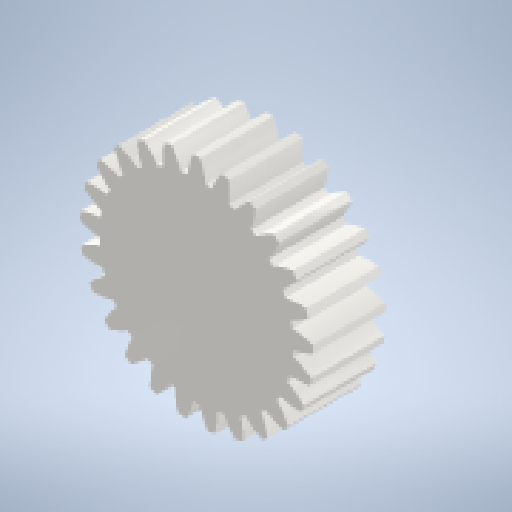
# Autodesk Inventor part: Spur Gear1
Saved by Autodesk Inventor 2023 (Build 270158030, 158C)
## iProperties
Created: 2024-09-26
Part Number: Spur Gear1
Material: Steel
Document SubType Name: Modeling
Designer: lvrectanus0
Categories: <?xml version="1.0" encoding="UTF-16"?> <MemberInstance><Categories><FamilyTemplate><FamilyTemplateParameter ValueType="xs:double" Id="1" ObjectReferenceKey="da_z" ObjectType="kUserParameterObject"/><FamilyTemplateParameter ValueType="xs:double" Id="2" ObjectReferenceKey="da_b" ObjectType="kUserParameterObject"/><FamilyTemplateParameter ValueType="xs:double" Id="3" ObjectReferenceKey="da_beta" ObjectType="kUserParameterObject"/><FamilyTemplateParameter ValueType="xs:double" Id="4" ObjectReferenceKey="da_da" ObjectType="kUserParameterObject"/><FamilyTemplateParameter ValueType="xs:double" Id="5" ObjectReferenceKey="da_aw" ObjectType="kUserParameterObject"/><FamilyTemplateParameter ValueType="xs:string" Id="6" ObjectReferenceKey="EAIAABAAAAC/AAAAAAAAAIAAAAAAAAAA" ObjectType="83910656" SubObjectId="SurfaceGeometry"/></FamilyTemplate><ParamToTemplateMap><ParamToTemplate CategoryParameter="//CategoryParameter[@InternalName='046C89C9-8512-4d59-83FE-43B91F4F132A']" TemplateParameter="1"/><ParamToTemplate CategoryParameter="//CategoryParameter[@InternalName='2552DF32-E462-4b46-AEBF-C6C7768E72AC']" TemplateParameter="2"/><ParamToTemplate CategoryParameter="//CategoryParameter[@InternalName='C9EE641D-15FC-4fae-A226-E94C4372FDD7']" TemplateParameter="3"/><ParamToTemplate><ParamToTemplate CategoryParameter="//CategoryParameter[@InternalName='00B6519A-459B-49c7-AD84-2E56D39A5744']" ConstantValue="0.000000"/></ParamToTemplate><ParamToTemplate><ParamToTemplate CategoryParameter="//CategoryParameter[@InternalName='04B31F0E-C7A6-4894-AA32-9629BEFACF47']" ConstantValue="1.000000"/></ParamToTemplate><ParamToTemplate><ParamToTemplate CategoryParameter="//CategoryParameter[@InternalName='43CBEC2E-7847-49e7-A936-2F7889FCB2D9']" ConstantValue="0.250000"/></ParamToTemplate><ParamToTemplate><ParamToTemplate CategoryParameter="//CategoryParameter[@InternalName='B1EFC894-105D-4ebd-86BF-FA20ED196853']" ConstantValue="0.350000"/></ParamToTemplate><ParamToTemplate><ParamToTemplate CategoryParameter="//CategoryParameter[@InternalName='51175063-3D10-4879-93E8-6246FE8B403D']" ConstantValue="2061532430.657340"/></ParamToTemplate><ParamToTemplate><ParamToTemplate CategoryParameter="//CategoryParameter[@InternalName='A3A52E27-4454-46a9-B0BD-C932399B70AF']" ConstantValue="0.300000"/></ParamToTemplate><ParamToTemplate><ParamToTemplate CategoryParameter="//CategoryParameter[@InternalName='91B76062-C214-41d9-B1B9-14D2AB99603D']" ConstantValue="0.149412"/></ParamToTemplate><ParamToTemplate><ParamToTemplate CategoryParameter="//CategoryParameter[@InternalName='374E806E-8B8A-4dda-A9AA-1039D6500AD2']" ConstantValue="6.692913"/></ParamToTemplate><ParamToTemplate><ParamToTemplate CategoryParameter="//CategoryParameter[@InternalName='2D373A89-B862-43d6-8D0B-0CBF12AB9F6C']" ConstantValue="0.349066"/></ParamToTemplate><ParamToTemplate CategoryParameter="//CategoryParameter[@InternalName='37777632-D6A2-4fac-9D53-DB8ACD95C989']" TemplateParameter="4"/><ParamToTemplate CategoryParameter="//CategoryParameter[@InternalName='FD1017F1-B727-4f7e-9707-0F86F1FF9423']" TemplateParameter="5"/><ParamToTemplate><ParamToTemplate CategoryParameter="//CategoryParameter[@InternalName='9E1B4470-B2D3-4ff1-B813-535BB4CDF51A']" ConstantValue="3523220.976809"/></ParamToTemplate><ParamToTemplate><ParamToTemplate CategoryParameter="//CategoryParameter[@InternalName='F8452263-BFF6-458c-9FB1-07C4B99E95CD']" ConstantValue="11397033.805607"/></ParamToTemplate><ParamToTemplate><ParamToTemplate CategoryParameter="//CategoryParameter[@InternalName='3E3BB259-FD49-497f-8171-6EBC954A3479']" ConstantValue="2.000000"/></ParamToTemplate><ParamToTemplate CategoryParameter="//CategoryParameter[@InternalName='27C3BAF2-7550-4e4b-AE2C-0DB134B7D9B7']" TemplateParameter="6"/></ParamToTemplateMap><Category DisplayName="Gear" InternalName="DC85795E-93AB-48d5-8EEE-5A27447B64BD" Mnemonic="Gear"><CategoryParameter DisplayName="z" InternalName="046C89C9-8512-4d59-83FE-43B91F4F132A" Mnemonic="z"/><CategoryParameter DisplayName="b" InternalName="2552DF32-E462-4b46-AEBF-C6C7768E72AC" Mnemonic="b"/><CategoryParameter DisplayName="||b|" InternalName="C9EE641D-15FC-4fae-A226-E94C4372FDD7" Mnemonic="beta"/><CategoryParameter DisplayName="x" InternalName="00B6519A-459B-49c7-AD84-2E56D39A5744" Mnemonic="x"/><CategoryParameter DisplayName="a*" InternalName="04B31F0E-C7A6-4894-AA32-9629BEFACF47" Mnemonic="a"/><CategoryParameter DisplayName="c*" InternalName="43CBEC2E-7847-49e7-A936-2F7889FCB2D9" Mnemonic="c"/><CategoryParameter DisplayName="r|.f|*" InternalName="B1EFC894-105D-4ebd-86BF-FA20ED196853" Mnemonic="rf"/><CategoryParameter DisplayName="E" InternalName="51175063-3D10-4879-93E8-6246FE8B403D" Mnemonic="E"/><CategoryParameter DisplayName="||m|" InternalName="A3A52E27-4454-46a9-B0BD-C932399B70AF" Mnemonic="mi"/><Category DisplayName="SpurGear" InternalName="26C5A22E-A91E-4dfd-A3B3-23CCAFAE1764" Mnemonic="SpurGear"><CategoryParameter DisplayName="m" InternalName="91B76062-C214-41d9-B1B9-14D2AB99603D" Mnemonic="m"/><CategoryParameter DisplayName="P" InternalName="374E806E-8B8A-4dda-A9AA-1039D6500AD2" Mnemonic="PP"/><CategoryParameter DisplayName="||a|" InternalName="2D373A89-B862-43d6-8D0B-0CBF12AB9F6C" Mnemonic="alpha"/><CategoryParameter DisplayName="d|.a|" InternalName="37777632-D6A2-4fac-9D53-DB8ACD95C989" Mnemonic="da"/><CategoryParameter DisplayName="a|.w|" InternalName="FD1017F1-B727-4f7e-9707-0F86F1FF9423" Mnemonic="aw"/><CategoryParameter DisplayName="||s||.Flim|" InternalName="9E1B4470-B2D3-4ff1-B813-535BB4CDF51A" Mnemonic="sFlim"/><CategoryParameter DisplayName="||s||.Hlim|" InternalName="F8452263-BFF6-458c-9FB1-07C4B99E95CD" Mnemonic="sHlim"/><CategoryParameter DisplayName="type" InternalName="3E3BB259-FD49-497f-8171-6EBC954A3479" Mnemonic="type"/><CategoryParameter DisplayName="PitchDiameter" InternalName="27C3BAF2-7550-4e4b-AE2C-0DB134B7D9B7" Mnemonic="IDS_PITCHDIAM"/></Category></Category></Categories></MemberInstance>
Density: 1 g/cm^3
Appearance: Steel
CustomPartVersion: 1
Author: lvrectanus0
Autodesk Inventor part; units mm, degrees
ref_plane "YZ Plane" through (0, 0, 0) normal (1, 0, 0) x (0, 1, 0)
ref_plane "XZ Plane" through (0, 0, 0) normal (0, 1, 0) x (-1, 0, 0)
ref_plane "XY Plane" through (0, 0, 0) normal (0, 0, 1) x (1, 0, 0)
sketch "Sketch1" plane through (0, 0, 0) normal (0, 0, 1) x (1, 0, 0)
  circle A0 centre (0, 0) radius 20.1697
  dimension "d0" = 40.3394
  constraints: 1 centre point
  measures "d0" diameter of A0
extrude "Extrusion1" add sketch "Sketch1" along normal blind 12.7
sketch "Sketch2" plane through (0, 0, 0) normal (0, 0, -1) x (-1, 0, 0)
  circle A0 centre (0, 0) radius 20.1697 projected
  circle A1 centre (0, 0) radius 18.6765
  dimension "d3" = 37.3529
  constraints: 1 centre point, 1 coincident
  measures "d3" diameter of A1
surface extrude "Pitch Diameter" sketch "Sketch2" against normal through all shown no curves A1
ref_plane "Work Plane1" through (0, 0, 0) normal (1, 0, 0) x (0, 1, 0)
ref_plane "Work Plane2" through (0, 0, 0) normal (0.9921147, 0.1253332, 0) x (0, 0, 1)
ref_plane "Work Plane3" through (0, 0, 6.35) normal (0, 0, -1) x (-1, 0, 0)
spur gear teeth "Spur Gear" teeth 25 pitch diameter 37.3529 tip diameter 40.3394 root diameter 33.6176 face width 12.7 start plane through (0, 0, 0) normal (0, 0, -1) x (-1, 0, 0)
sketch "Sketch3" plane through (0, 0, 0) normal (0, 0, -1) x (-1, 0, 0)
  spline S0 degree 3 poles (13.7795, 0) (13.7795, 0.8167) (13.7075, 1.6265) (13.5636, 2.4297) (13.559, 2.4556) (13.5545, 2.4799) (13.5495, 2.5074) (13.392, 3.3584) (13.1564, 4.1874) (12.8426, 4.9942) (12.8325, 5.0202) (12.8227, 5.0451) (12.812, 5.0722) (12.4908, 5.8837) (12.0961, 6.6575) (11.628, 7.3936) (11.5968, 7.4426) (11.5659, 7.4905) (11.5334, 7.5403) (11.0131, 8.3362) (10.416, 9.0712) (9.7436, 9.7436) (9.1132, 10.374) (8.4283, 10.9377) (7.6889, 11.4348) (7.6396, 11.468) (7.589, 11.5015) (7.5403, 11.5334) (6.7854, 12.0269) (5.9898, 12.4423) (5.1532, 12.7796) (5.1263, 12.7905) (5.0981, 12.8017) (5.0722, 12.812) (4.2674, 13.1306) (3.44, 13.3713) (2.5897, 13.534) (2.5623, 13.5392) (2.5332, 13.5447) (2.5074, 13.5495) (1.679, 13.7028) (0.8425, 13.7795) (0, 13.7795) (-0.8161, 13.7795) (-1.626, 13.7076) (-2.4296, 13.5636) (-2.4555, 13.559) (-2.4799, 13.5545) (-2.5074, 13.5495) (-3.3584, 13.392) (-4.1874, 13.1564) (-4.9942, 12.8426) (-5.0202, 12.8325) (-5.0451, 12.8227) (-5.0722, 12.812) (-5.8837, 12.4908) (-6.6575, 12.0961) (-7.3936, 11.628) (-7.4426, 11.5968) (-7.4905, 11.5659) (-7.5403, 11.5334) (-8.3362, 11.0131) (-9.0712, 10.416) (-9.7436, 9.7436) (-10.374, 9.1132) (-10.9377, 8.4283) (-11.4348, 7.6889) (-11.468, 7.6396) (-11.5015, 7.589) (-11.5334, 7.5403) (-12.0269, 6.7854) (-12.4423, 5.9898) (-12.7796, 5.1532) (-12.7905, 5.1263) (-12.8017, 5.0981) (-12.812, 5.0722) (-13.1306, 4.2674) (-13.3713, 3.44) (-13.534, 2.5897) (-13.5392, 2.5623) (-13.5447, 2.5332) (-13.5495, 2.5074) (-13.7028, 1.679) (-13.7795, 0.8425) (-13.7795, 0) knots 0 0 0 0 0.030273 0.030273 0.030273 0.03125 0.03125 0.03125 0.061523 0.061523 0.061523 0.0625 0.0625 0.0625 0.091797 0.091797 0.091797 0.09375 0.09375 0.09375 0.125 0.125 0.125 0.154297 0.154297 0.154297 0.15625 0.15625 0.15625 0.186523 0.186523 0.186523 0.1875 0.1875 0.1875 0.217773 0.217773 0.217773 0.21875 0.21875 0.21875 0.25 0.25 0.25 0.280273 0.280273 0.280273 0.28125 0.28125 0.28125 0.311523 0.311523 0.311523 0.3125 0.3125 0.3125 0.341797 0.341797 0.341797 0.34375 0.34375 0.34375 0.375 0.375 0.375 0.404297 0.404297 0.404297 0.40625 0.40625 0.40625 0.436523 0.436523 0.436523 0.4375 0.4375 0.4375 0.467773 0.467773 0.467773 0.46875 0.46875 0.46875 0.5 0.5 0.5 0.5 projected
  spline S1 degree 3 poles (-13.7795, 0) (-13.7795, -0.8161) (-13.7076, -1.626) (-13.5636, -2.4296) (-13.559, -2.4555) (-13.5545, -2.4799) (-13.5495, -2.5074) (-13.392, -3.3584) (-13.1564, -4.1874) (-12.8426, -4.9942) (-12.8325, -5.0202) (-12.8227, -5.0451) (-12.812, -5.0722) (-12.4908, -5.8837) (-12.0961, -6.6575) (-11.628, -7.3936) (-11.5968, -7.4426) (-11.5659, -7.4905) (-11.5334, -7.5403) (-11.0131, -8.3362) (-10.416, -9.0712) (-9.7436, -9.7436) (-9.1132, -10.374) (-8.4283, -10.9377) (-7.6889, -11.4348) (-7.6396, -11.468) (-7.589, -11.5015) (-7.5403, -11.5334) (-6.7854, -12.0269) (-5.9898, -12.4423) (-5.1532, -12.7796) (-5.1263, -12.7905) (-5.0981, -12.8017) (-5.0722, -12.812) (-4.2674, -13.1306) (-3.44, -13.3713) (-2.5897, -13.534) (-2.5623, -13.5392) (-2.5332, -13.5447) (-2.5074, -13.5495) (-1.679, -13.7028) (-0.8425, -13.7795) (0, -13.7795) (0.8161, -13.7795) (1.626, -13.7076) (2.4296, -13.5636) (2.4555, -13.559) (2.4799, -13.5545) (2.5074, -13.5495) (3.3584, -13.392) (4.1874, -13.1564) (4.9942, -12.8426) (5.0202, -12.8325) (5.0451, -12.8227) (5.0722, -12.812) (5.8837, -12.4908) (6.6575, -12.0961) (7.3936, -11.628) (7.4426, -11.5968) (7.4905, -11.5659) (7.5403, -11.5334) (8.3362, -11.0131) (9.0712, -10.416) (9.7436, -9.7436) (10.374, -9.1132) (10.9377, -8.4283) (11.4348, -7.6889) (11.468, -7.6396) (11.5015, -7.589) (11.5334, -7.5403) (12.0269, -6.7854) (12.4423, -5.9898) (12.7796, -5.1532) (12.7905, -5.1263) (12.8017, -5.0981) (12.812, -5.0722) (13.1306, -4.2674) (13.3713, -3.44) (13.534, -2.5897) (13.5392, -2.5623) (13.5447, -2.5333) (13.5495, -2.5074) (13.7029, -1.6784) (13.7796, -0.8426) (13.7795, 0) knots 0.5 0.5 0.5 0.5 0.530273 0.530273 0.530273 0.53125 0.53125 0.53125 0.561523 0.561523 0.561523 0.5625 0.5625 0.5625 0.591797 0.591797 0.591797 0.59375 0.59375 0.59375 0.625 0.625 0.625 0.654297 0.654297 0.654297 0.65625 0.65625 0.65625 0.686523 0.686523 0.686523 0.6875 0.6875 0.6875 0.717773 0.717773 0.717773 0.71875 0.71875 0.71875 0.75 0.75 0.75 0.780273 0.780273 0.780273 0.78125 0.78125 0.78125 0.811523 0.811523 0.811523 0.8125 0.8125 0.8125 0.841797 0.841797 0.841797 0.84375 0.84375 0.84375 0.875 0.875 0.875 0.904297 0.904297 0.904297 0.90625 0.90625 0.90625 0.936523 0.936523 0.936523 0.9375 0.9375 0.9375 0.967773 0.967773 0.967773 0.96875 0.96875 0.96875 1 1 1 1 projected
  line L0 (-2.7496, 4.7625) -> (2.7496, 4.7625) projected
  line L1 (2.7496, 4.7625) -> (5.4993, 0) projected
  line L2 (5.4993, 0) -> (2.7496, -4.7625) projected
  line L3 (2.7496, -4.7625) -> (-2.7496, -4.7625) projected
  line L4 (-2.7496, -4.7625) -> (-5.4993, 0) projected
  line L5 (-5.4993, 0) -> (-2.7496, 4.7625) projected
  point P0 (0, 0)
ref_plane "Work Plane4" through (-13.7797, -13.7797, -7.9273) normal (0, 0, -1) x (0, 1, 0)
extrude "Extrusion2" add sketch "Sketch3" along normal up to surface (7.9273 mm away) contours L0 L1 L2 L3 L4 L5
chamfer "Chamfer1" distance 1.27 angle 45 6 edges at (4.1244, 2.3813, -7.9273) (0, 4.7625, -7.9273) (-4.1244, 2.3813, -7.9273) (-4.1244, -2.3813, -7.9273) (0, -4.7625, -7.9273) (4.1244, -2.3813, -7.9273)
equation "\"d0\" = da_da"
equation "\"d1\" = da_b"
equation "\"d3\" = da_d"
equation "\"d15\" = da_aw"
equation "\"d19\" = da_aw"
equation "\"da_da\" = 40.339364"
equation "\"da_b\" = 12.7"
equation "\"da_d\" = 37.352941"
equation "\"da_aw\" = 47.171429"
body "Solid1"
body "Srf1"
